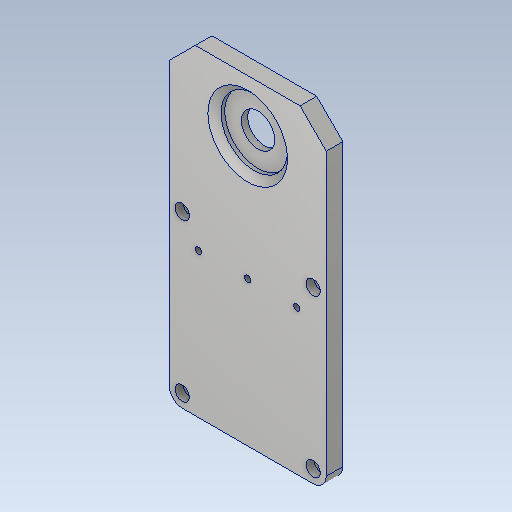
# Autodesk Inventor part: FAB-P0041 - Camera Support Plate V2
Saved by Autodesk Inventor 2020 (Build 240168000, 168)
## iProperties
Created: 2012-07-23
Part Number: FAB-P0041 - Camera Support Plate V2
Material: Aluminum 6061
Document SubType Name: Modeling
Designer: map
Density: 2.7 g/cm^3
Appearance: Aluminum - Flat
Mass: 940.783 g
Surface Area: 695.863 cm^2
Volume: 348.438 cm^3
Sending System: SolidWorks 2015
Last Author: ml2377
Last Saved: 2016-03-24
Author: map
Autodesk Inventor part; units mm, degrees
ref_plane "XZ Plane" through (0, 0, 0) normal (0, 1, 0) x (-1, 0, 0)
ref_plane "XY Plane" through (0, 0, 0) normal (0, 0, 1) x (1, 0, 0)
derived "__05_Detection_MASTER__.ipt"
sketch "Sketch1_1" plane through (0, 0, 0) normal (0, 0, 1) x (1, 0, 0)
  line L0 (-119.8204, -325) -> (119.8204, -325)
  line L1 (0, 0) -> (0, -325) construction
  line L2 (-50, -75) -> (50, -75)
  line L3 (50, -75) -> (50, -195)
  line L4 (50, -195) -> (-50, -195)
  line L5 (-50, -195) -> (-50, -75)
  line L6 (-22.9, -88) -> (114.26, -88)
  line L7 (-37.5, -94.5) -> (37.5, -94.5)
  line L8 (-40.82, -88) -> (132.18, -88) construction
  point P0 (0, -75)
  point P1 (0, -94.5)
  point P2 (0, -94.5)
  point P3 (45.68, -88)
ref_plane "Work Plane1" through (-59.525, 0, 0) normal (1, 0, 0) x (0, 1, 0)
sketch "Sketch1" plane through (0, 0, 0) normal (1, 0, 0) x (0, 1, 0)
  line L0 (40, 0) -> (-205, 0)
  line L1 (40, -12.7) -> (40, 0)
  line L2 (-205, 0) -> (-205, -12.7)
  line L3 (40, -12.7) -> (-205, -12.7)
  line L4 (-75, 0) -> (-195, 0)
  point P0 (0, 0)
  dimension "d65" = 245
  dimension "d66" = 12.7
  dimension "d67" = 40
  dimension "d91" = 10
  constraints: 10 end point, 2 horizontal, 2 vertical, 1 collinear
  measures "d65" distance of L0.start L0.end
  measures "d66" distance of L0.end L2.end
  measures "d67" distance from line of point (0, 0) L1
  measures "d91" distance from line of L4.end L2
extrude "Extrusion1" add sketch "Sketch1" along normal mid plane 120
sketch "Sketch8" plane through (-60, -205, 0) normal (0, 0, 1) x (1, 0, 0)
  point P0 (60, 205)
  point P1 (60, 205)
  constraints: 1 coincident
hole "CMount" at (0, 0, 0) direction (0, 0, -1) diameter 25.4254 depth 12.7 counterbore diameter 50.8 counterbore depth 7.8994
sketch "Sketch7" plane through (-60, -205, 0) normal (0, 0, 1) x (1, 0, 0)
  line L0 (10, 130) -> (110, 130) projected
  line L1 (10, 10) -> (10, 130) projected
  line L2 (110, 10) -> (10, 10) projected
  line L3 (110, 130) -> (110, 10) projected
  constraints: 3 coincident
hole "M6CBore" at (50, -195, 0) at (-50, -75, 0) at (50, -75, 0) at (-50, -195, 0) direction (0, 0, -1) diameter 6.4 depth 12.7 counterbore diameter 11 counterbore depth 6.1
chamfer "Chamfer3" distance 5 angle 45 1 edges at (0, 25.4, 0)
chamfer "Chamfer2" distance 20 angle 45 1 edges at (60, 40, -6.35)
chamfer "Chamfer1" distance 20 angle 45 1 edges at (-60, 40, -6.35)
hole "Hole12" at (37.5, -94.5, 0) at (0, -94.5, 0) at (-37.5, -94.5, 0) direction (0, 0, -1) diameter 4.917 end through all thread size "M6x1" class "6H" standard "ISO Metric profile"
fillet "Fillet1" radius 10 2 edges at (-60, -205, -6.35) (60, -205, -6.35)
body "Solid3"
